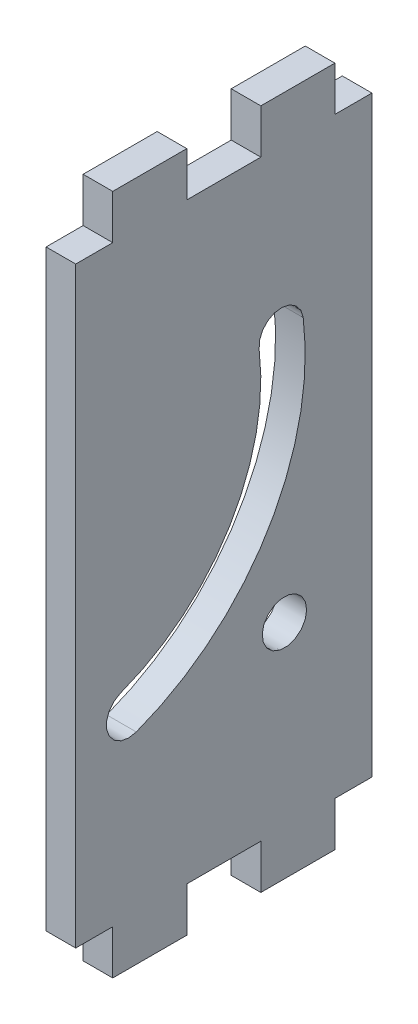
# Autodesk Inventor part: side.plate.cam.rev3
Saved by Autodesk Inventor 2025.2 (Build 292293000, 293)
## iProperties
Created: 2016-03-08
Part Number: side.plate.cam.rev3
Material: 一般
Document SubType Name: Modeling
Designer: 200288284
Density: 1 g/cm^3
Appearance: 默认值
Author: 200288284
Autodesk Inventor part; units mm, degrees
ref_plane "YZ Plane" through (0, 0, 0) normal (1, 0, 0) x (0, 1, 0)
ref_plane "XZ Plane" through (0, 0, 0) normal (0, 1, 0) x (-1, 0, 0)
ref_plane "XY Plane" through (0, 0, 0) normal (0, 0, 1) x (1, 0, 0)
sketch "Sketch1" plane through (0, 0, 0) normal (1, 0, 0) x (0, 1, 0)
  line L0 (0, 20) -> (-40, 20)
  line L1 (-40, 0) -> (0, 0)
  line L2 (3, 7.5) -> (0, 7.5)
  line L3 (3, 7.5) -> (3, 2.5)
  line L4 (3, 2.5) -> (0, 2.5)
  circle A0 centre (-28, 5.9065) radius 1.5
  arc A1 (-26.5938, 16.9542) -> (-29.4062, 15.9103) centre (-28, 16.4322) ccw
  arc A2 (-10.8125, 4.6373) -> (-11.1875, 7.6137) centre (-11, 6.1255) ccw
  arc A3 (-26.5938, 16.9542) -> (-11.1875, 7.6137) centre (-13, 22) ccw
  arc A4 (-29.4062, 15.9103) -> (-10.8125, 4.6373) centre (-13, 22) ccw
  line L5 (0, 0) -> (0, 20)
  line L6 (-40, 0) -> (-40, 20)
  line L7 (0, 2.5) -> (0, 7.5)
  line L8 (0, 10) -> (-40, 10)
  line L9 (-28, 5.9065) -> (-28, 16.4322)
  line L10 (-11, 6.1255) -> (-28, 6.1255)
  line L11 (3, 12.5) -> (0, 12.5)
  line L12 (3, 12.5) -> (3, 17.5)
  line L13 (3, 17.5) -> (0, 17.5)
  line L14 (-20, 0) -> (-20, 20)
  line L15 (-43, 7.5) -> (-40, 7.5)
  line L16 (-43, 7.5) -> (-43, 2.5)
  line L17 (-43, 2.5) -> (-40, 2.5)
  line L18 (-43, 12.5) -> (-43, 17.5)
  line L19 (-43, 17.5) -> (-40, 17.5)
  line L20 (-43, 12.5) -> (-40, 12.5)
  point P0 (0, 12.5)
  point P1 (0, 17.5)
  point P2 (-20, 10)
  point P3 (-20, 9.3016)
  point P4 (-20.3655, 6.1255)
  point P5 (-26.5161, 6.1255)
  point P6 (-28, 7.4065)
  point P7 (-28, 12.9861)
  point P8 (-21.1394, 10)
  dimension "d9" = 3
  dimension "d11" = 3
  dimension "d12" = 3
  dimension "d16" = 20
  dimension "d17" = 40
  dimension "d18" = 5
  dimension "d19" = 3
  dimension "d20" = 14.5
  dimension "d21" = 17.5
  dimension "d22" = 22
  dimension "d23" = 13
  dimension "d24" = 22
  dimension "d26" = 15
  dimension "d27" = 17
  dimension "d28" = 2.5
  constraints: 42 end point, 12 point on circle, 12 symmetric about line, 5 centre point, 4 midpoint, 3 perpendicular, 3 vertical, 2 coincident, 1 collinear, 1 horizontal, 1 parallel, 1 point on line
  measures "d9" diameter of A0
  measures "d11" diameter of A1
  measures "d12" diameter of A2
  measures "d16" distance between parallel lines of L0 L1
  measures "d17" distance between parallel lines of L6 L5
  measures "d18" distance between parallel lines of L2 L4
  measures "d19" distance between parallel lines of L7 L3
  measures "d20" radius of A3
  measures "d21" radius of A4
  measures "d22" distance of A3.centre L9.start
  measures "d23" horizontal distance of point (0, 0) A4.centre
  measures "d24" vertical distance of point (0, 0) A4.centre
  measures "d26" horizontal distance of A3.centre L9.end
  measures "d27" distance of L10.start L10.end
  measures "d28" distance between parallel lines of L8 L2
extrude "Extrusion1" add sketch "Sketch1" along normal blind 2 contours L5 L8 L14 L0 | L14 L8 A3 A1 A4 L9 L6 L0 | L13 L12 L11 L5 | L14 A3 L8 | L8 L5 L1 L14 A4 A2 A3 | L6 L20 L18 L19 | L2 L3 L4 L5 | L8 L9 A4 | A4 L10 A0 L9 L8 | L8 L9 A0 L10 A4 L14 L1 L6 | L6 L17 L16 L15
body "Solid1"
